Autodesk Fusion 360 part; units mm, degrees
note: some values were not read from the file. Chosen so that the rebuilt part matches the saved one: which face or edge a step refers to. Set by a fixed rule: which sketch regions a step uses.
(part 2 of 2)
sketch "Sketch4" plane through (20.4456, 0, 0) normal (1, 0, 0) x (0, 0, -1)
  arc A0 (20.4324, 154.945) -> (19.9602, 157.428) centre (20.32, 156.21) ccw
  arc A1 (19.9602, 157.428) -> (20.4324, 154.945) centre (20.0726, 156.1629) ccw
  circle A2 centre (21.6948, 142.2077) radius 3.175
  line L0 (12.648, 144.8633) -> (12.648, 132.4457)
  line L1 (12.648, 132.4457) -> (10.108, 132.4457)
  line L2 (10.108, 132.4457) -> (10.108, 144.8633)
  line L3 (10.108, 144.8633) -> (12.648, 144.8633)
  line L4 (-81.332, 144.78) -> (-78.792, 144.78)
  line L5 (-78.792, 144.78) -> (-78.792, 138.684)
  line L6 (-78.792, 138.684) -> (-81.332, 138.684)
  line L7 (-81.332, 138.684) -> (-81.332, 144.78)
  circle A3 centre (-84.1517, 161.0274) radius 3.175
  circle A4 centre (24.5119, 159.7522) radius 3.175
  arc A5 (-20.372, 13.97) -> (-12.752, 6.35) centre (-12.752, 13.97) ccw
  line L8 (-20.372, 13.97) -> (-20.372, 54.61)
  arc A6 (-20.372, 54.61) -> (-27.992, 62.23) centre (-27.992, 54.61) ccw
  line L9 (-27.992, 62.23) -> (-41.962, 62.23)
  arc A7 (-49.582, 69.85) -> (-41.962, 62.23) centre (-41.962, 69.85) ccw
  line L10 (-49.582, 69.85) -> (-49.582, 113.03)
  arc A8 (-41.962, 120.65) -> (-49.582, 113.03) centre (-41.962, 113.03) ccw
  line L11 (-41.962, 120.65) -> (-27.992, 120.65)
  arc A9 (-27.992, 120.65) -> (-20.372, 128.27) centre (-27.992, 128.27) ccw
  line L12 (-20.372, 128.27) -> (-20.372, 132.08)
  arc A10 (-12.752, 139.7) -> (-20.372, 132.08) centre (-12.752, 132.08) ccw
  line L13 (-12.752, 139.7) -> (-1.322, 139.7)
  arc A11 (6.298, 132.08) -> (-1.322, 139.7) centre (-1.322, 132.08) ccw
  line L14 (6.298, 132.08) -> (6.298, 13.97)
  arc A12 (-1.322, 6.35) -> (6.298, 13.97) centre (-1.322, 13.97) ccw
  line L15 (-1.322, 6.35) -> (-12.752, 6.35)
  line L16 (-18.467, 0) -> (-18.467, -2.54)
  line L17 (-18.467, -2.54) -> (3.4968, -2.54)
  line L18 (3.4968, -2.54) -> (3.4968, -10.16)
  line L19 (3.4968, -10.16) -> (10.108, -10.16)
  line L20 (10.108, -10.16) -> (10.108, -2.54)
  line L21 (10.108, -2.54) -> (12.648, -2.54)
  line L22 (12.648, -2.54) -> (12.648, -10.16)
  line L23 (12.648, -10.16) -> (20.32, -10.16)
  line L24 (20.32, -10.16) -> (20.32, 124.46)
  line L25 (20.32, 124.46) -> (30.428, 124.46)
  line L26 (30.428, 124.46) -> (30.428, 165.1009)
  line L27 (30.428, 165.1009) -> (17.232, 165.1009)
  arc A13 (18.014, 152.4) -> (17.232, 165.1009) centre (-85.5242, 152.4) ccw
  line L28 (18.014, 152.4) -> (-21.642, 152.4)
  line L29 (-21.642, 152.4) -> (-21.642, 145.288)
  line L30 (-21.642, 145.288) -> (-24.182, 145.288)
  line L31 (-24.182, 145.288) -> (-24.182, 152.4)
  line L32 (-24.182, 152.4) -> (-81.332, 152.4)
  line L33 (-81.332, 152.4) -> (-81.332, 152.4009)
  line L34 (-81.332, 152.4009) -> (-86.7309, 152.4009)
  line L35 (-86.7309, 152.4009) -> (-87.0413, 154.9409)
  line L36 (-87.0413, 154.9409) -> (-73.712, 156.5697)
  line L37 (-73.712, 156.5697) -> (-73.712, 166.37)
  line L38 (-73.712, 166.37) -> (-94.032, 166.37)
  line L39 (-94.032, 166.37) -> (-94.032, 127.3528)
  line L40 (-94.032, 127.3528) -> (-81.332, 127.3528)
  line L41 (-81.332, 127.3528) -> (-81.332, 12.7)
  line L42 (-81.332, 12.7) -> (-91.44, 12.7)
  line L43 (-91.44, 12.7) -> (-91.44, -10.16)
  line L44 (-91.44, -10.16) -> (-81.332, -10.16)
  line L45 (-81.332, -10.16) -> (-81.332, -2.54)
  line L46 (-81.332, -2.54) -> (-78.792, -2.54)
  line L47 (-78.792, -2.54) -> (-78.792, -10.16)
  line L48 (-78.792, -10.16) -> (-63.5, -10.16)
  line L49 (-63.5, -10.16) -> (-63.5, -2.54)
  line L50 (-63.5, -2.54) -> (-34.215, -2.54)
  line L51 (-34.215, -2.54) -> (-34.215, 0)
  line L52 (-34.215, 0) -> (-18.467, 0)
  arc A14 (20.4324, 154.945) -> (19.9602, 157.428) centre (20.32, 156.21) ccw
  arc A15 (19.9602, 157.428) -> (20.4324, 154.945) centre (20.0726, 156.1629) ccw
  circle A16 centre (21.6948, 142.2077) radius 3.175
  line L53 (12.648, 132.4457) -> (12.648, 144.8633)
  line L54 (12.648, 144.8633) -> (10.108, 144.8633)
  line L55 (10.108, 144.8633) -> (10.108, 132.4457)
  line L56 (10.108, 132.4457) -> (12.648, 132.4457)
  line L57 (-78.792, 144.78) -> (-81.332, 144.78)
  line L58 (-81.332, 144.78) -> (-81.332, 138.684)
  line L59 (-81.332, 138.684) -> (-78.792, 138.684)
  line L60 (-78.792, 138.684) -> (-78.792, 144.78)
  circle A17 centre (-84.1517, 161.0274) radius 3.175
  circle A18 centre (24.5119, 159.7522) radius 3.175
  arc A19 (-20.372, 13.97) -> (-12.752, 6.35) centre (-12.752, 13.97) ccw
  line L61 (-12.752, 6.35) -> (-1.322, 6.35)
  arc A20 (-1.322, 6.35) -> (6.298, 13.97) centre (-1.322, 13.97) ccw
  line L62 (6.298, 13.97) -> (6.298, 132.08)
  arc A21 (6.298, 132.08) -> (-1.322, 139.7) centre (-1.322, 132.08) ccw
  line L63 (-1.322, 139.7) -> (-12.752, 139.7)
  arc A22 (-12.752, 139.7) -> (-20.372, 132.08) centre (-12.752, 132.08) ccw
  line L64 (-20.372, 132.08) -> (-20.372, 128.27)
  arc A23 (-27.992, 120.65) -> (-20.372, 128.27) centre (-27.992, 128.27) ccw
  line L65 (-27.992, 120.65) -> (-41.962, 120.65)
  arc A24 (-41.962, 120.65) -> (-49.582, 113.03) centre (-41.962, 113.03) ccw
  line L66 (-49.582, 113.03) -> (-49.582, 69.85)
  arc A25 (-49.582, 69.85) -> (-41.962, 62.23) centre (-41.962, 69.85) ccw
  line L67 (-41.962, 62.23) -> (-27.992, 62.23)
  arc A26 (-20.372, 54.61) -> (-27.992, 62.23) centre (-27.992, 54.61) ccw
  line L68 (-20.372, 54.61) -> (-20.372, 13.97)
  line L69 (-18.467, -2.54) -> (-18.467, 0)
  line L70 (-18.467, 0) -> (-34.215, 0)
  line L71 (-34.215, 0) -> (-34.215, -2.54)
  line L72 (-34.215, -2.54) -> (-63.5, -2.54)
  line L73 (-63.5, -2.54) -> (-63.5, -10.16)
  line L74 (-63.5, -10.16) -> (-78.792, -10.16)
  line L75 (-78.792, -10.16) -> (-78.792, -2.54)
  line L76 (-78.792, -2.54) -> (-81.332, -2.54)
  line L77 (-81.332, -2.54) -> (-81.332, -10.16)
  line L78 (-81.332, -10.16) -> (-91.44, -10.16)
  line L79 (-91.44, -10.16) -> (-91.44, 12.7)
  line L80 (-91.44, 12.7) -> (-81.332, 12.7)
  line L81 (-81.332, 12.7) -> (-81.332, 127.3528)
  line L82 (-81.332, 127.3528) -> (-94.032, 127.3528)
  line L83 (-94.032, 127.3528) -> (-94.032, 166.37)
  line L84 (-94.032, 166.37) -> (-73.712, 166.37)
  line L85 (-73.712, 166.37) -> (-73.712, 156.5697)
  line L86 (-73.712, 156.5697) -> (-87.0413, 154.9409)
  line L87 (-87.0413, 154.9409) -> (-86.7309, 152.4009)
  line L88 (-86.7309, 152.4009) -> (-81.332, 152.4009)
  line L89 (-81.332, 152.4009) -> (-81.332, 152.4)
  line L90 (-81.332, 152.4) -> (-24.182, 152.4)
  line L91 (-24.182, 152.4) -> (-24.182, 145.288)
  line L92 (-24.182, 145.288) -> (-21.642, 145.288)
  line L93 (-21.642, 145.288) -> (-21.642, 152.4)
  line L94 (-21.642, 152.4) -> (18.014, 152.4)
  arc A27 (18.014, 152.4) -> (17.232, 165.1009) centre (-85.5242, 152.4) ccw
  line L95 (17.232, 165.1009) -> (30.428, 165.1009)
  line L96 (30.428, 165.1009) -> (30.428, 124.46)
  line L97 (30.428, 124.46) -> (20.32, 124.46)
  line L98 (20.32, 124.46) -> (20.32, -10.16)
  line L99 (20.32, -10.16) -> (12.648, -10.16)
  line L100 (12.648, -10.16) -> (12.648, -2.54)
  line L101 (12.648, -2.54) -> (10.108, -2.54)
  line L102 (10.108, -2.54) -> (10.108, -10.16)
  line L103 (10.108, -10.16) -> (3.4968, -10.16)
  line L104 (3.4968, -10.16) -> (3.4968, -2.54)
  line L105 (3.4968, -2.54) -> (-18.467, -2.54)
  line L106 (-68.58, 144.78) -> (-58.42, 144.78)
  line L107 (-58.42, 144.78) -> (-58.42, 152.4)
  line L108 (-58.42, 152.4) -> (-68.58, 152.4)
  line L109 (-68.58, 152.4) -> (-68.58, 144.78)
  line L110 (-38.1, 144.78) -> (-30.48, 144.78)
  line L111 (-30.48, 144.78) -> (-30.48, 152.4)
  line L112 (-30.48, 152.4) -> (-38.1, 152.4)
  line L113 (-38.1, 152.4) -> (-38.1, 144.78)
  line L114 (3.3659, 148.59) -> (10.108, 148.59)
  line L115 (10.108, 148.59) -> (10.108, 152.4)
  line L116 (10.108, 152.4) -> (3.3659, 152.4)
  line L117 (3.3659, 152.4) -> (3.3659, 148.59)
  point P0 (10.108, 152.4)
extrude "Extrude4'" cut sketch "Sketch4" against normal blind 2.54 contours L28 L94 L114 L115 L116 L117 | L32 L90 L110 L111 L112 L113 | L32 L90 L106 L107 L108 L109 bodies 6 in component "right"
sketch "Sketch5" plane through (0, 0, -12.648) normal (0, 0, -1) x (-1, 0, 0)
  line L0 (39.2444, -2.54) -> (39.2444, 0)
  line L1 (39.2444, 0) -> (49.4044, 0)
  line L2 (49.4044, 0) -> (49.4044, -2.54)
  line L3 (49.4044, -2.54) -> (39.2444, -2.54)
  line L4 (-9.7776, -2.54) -> (-9.7776, 0)
  line L5 (-9.7776, 0) -> (3.4304, 0)
  line L6 (3.4304, 0) -> (3.4304, -2.54)
  line L7 (3.4304, -2.54) -> (-9.7776, -2.54)
  line L8 (64.6444, -2.54) -> (64.6444, 132.4457)
  line L9 (64.6444, 132.4457) -> (69.7244, 132.4457)
  line L10 (69.7244, 132.4457) -> (69.7244, 144.7757)
  arc A0 (69.7244, 144.7757) -> (64.6444, 144.8633) centre (64.6444, -2.54) ccw
  line L11 (64.6444, 144.8633) -> (64.6444, 152.4)
  line L12 (64.6444, 152.4) -> (-17.9056, 152.4)
  line L13 (-17.9056, 152.4) -> (-17.9056, 144.8633)
  arc A1 (-17.9056, 144.8633) -> (-22.9856, 144.7757) centre (-17.9056, -2.54) ccw
  line L14 (-22.9856, 144.7757) -> (-22.9856, 132.4457)
  line L15 (-22.9856, 132.4457) -> (-17.9056, 132.4457)
  line L16 (-17.9056, 132.4457) -> (-17.9056, -2.54)
  line L17 (-17.9056, -2.54) -> (-20.4456, -2.54)
  line L18 (-20.4456, -2.54) -> (-20.7288, 7.6202)
  line L19 (-20.7288, 7.6202) -> (-24.3812, 7.6202)
  line L20 (-24.3812, 7.6202) -> (-24.3812, -10.16)
  line L21 (-24.3812, -10.16) -> (71.12, -10.16)
  line L22 (71.12, -10.16) -> (71.12, 7.6202)
  line L23 (71.12, 7.6202) -> (67.4676, 7.6202)
  line L24 (67.4676, 7.6202) -> (67.1844, -2.54)
  line L25 (67.1844, -2.54) -> (64.6444, -2.54)
  line L26 (-9.8069, 146.05) -> (-2.54, 146.05)
  line L27 (-2.54, 146.05) -> (-2.54, 152.4)
  line L28 (-2.54, 152.4) -> (-9.8069, 152.4)
  line L29 (-9.8069, 152.4) -> (-9.8069, 146.05)
  line L30 (12.1172, 146.05) -> (17.78, 146.05)
  line L31 (17.78, 146.05) -> (17.78, 152.4)
  line L32 (17.78, 152.4) -> (12.1172, 152.4)
  line L33 (12.1172, 152.4) -> (12.1172, 146.05)
  line L34 (-17.9056, 152.4) -> (64.6444, 152.4)
  line L35 (40.7725, 146.05) -> (50.8, 146.05)
  line L36 (50.8, 146.05) -> (50.8, 152.4)
  line L37 (50.8, 152.4) -> (40.7725, 152.4)
  line L38 (40.7725, 152.4) -> (40.7725, 146.05)
extrude "Extrude2''" cut sketch "Sketch5" against normal blind 2.54 contours L12 L34 L35 L36 L37 L38 | L12 L30 L31 L32 L33 L34 | L12 L26 L27 L28 L29 L34 bodies 3 in component "back"
sketch "Sketch6" plane through (-67.1844, 0, 0) normal (-1, 0, 0) x (0, 0, 1)
  circle A0 centre (-24.5119, 159.7522) radius 3.175
  circle A1 centre (-21.6948, 142.2077) radius 3.175
  circle A2 centre (-20.32, 156.21) radius 1.27
  line L0 (78.792, 144.78) -> (81.332, 144.78)
  line L1 (81.332, 144.78) -> (81.332, 138.684)
  line L2 (81.332, 138.684) -> (78.792, 138.684)
  line L3 (78.792, 138.684) -> (78.792, 144.78)
  circle A3 centre (84.1517, 161.0274) radius 3.175
  line L4 (-12.648, 132.4457) -> (-12.648, 144.8633)
  line L5 (-12.648, 144.8633) -> (-10.108, 144.8633)
  line L6 (-10.108, 144.8633) -> (-10.108, 132.4457)
  line L7 (-10.108, 132.4457) -> (-12.648, 132.4457)
  line L8 (81.332, -2.54) -> (81.332, -10.16)
  line L9 (81.332, -10.16) -> (91.44, -10.16)
  line L10 (91.44, -10.16) -> (91.44, 12.7)
  line L11 (91.44, 12.7) -> (81.332, 12.7)
  line L12 (81.332, 12.7) -> (81.332, 127.3528)
  line L13 (81.332, 127.3528) -> (94.032, 127.3528)
  line L14 (94.032, 127.3528) -> (94.032, 166.37)
  line L15 (94.032, 166.37) -> (73.712, 166.37)
  line L16 (73.712, 166.37) -> (73.712, 156.5697)
  line L17 (73.712, 156.5697) -> (87.0413, 154.9409)
  line L18 (87.0413, 154.9409) -> (86.7309, 152.4009)
  line L19 (86.7309, 152.4009) -> (81.332, 152.4009)
  line L20 (81.332, 152.4009) -> (81.332, 152.4)
  line L21 (81.332, 152.4) -> (24.182, 152.4)
  line L22 (24.182, 152.4) -> (24.182, 145.288)
  line L23 (24.182, 145.288) -> (21.642, 145.288)
  line L24 (21.642, 145.288) -> (21.642, 152.4)
  line L25 (21.642, 152.4) -> (-18.014, 152.4)
  arc A4 (-17.232, 165.1009) -> (-18.014, 152.4) centre (85.5242, 152.4) ccw
  line L26 (-17.232, 165.1009) -> (-30.428, 165.1009)
  line L27 (-30.428, 165.1009) -> (-30.428, 124.46)
  line L28 (-30.428, 124.46) -> (-12.648, 124.46)
  line L29 (-12.648, 124.46) -> (-12.648, 10.16)
  line L30 (-12.648, 10.16) -> (-20.32, 10.16)
  line L31 (-20.32, 10.16) -> (-20.32, -10.16)
  line L32 (-20.32, -10.16) -> (-12.648, -10.16)
  line L33 (-12.648, -10.16) -> (-12.648, -2.54)
  line L34 (-12.648, -2.54) -> (-10.108, -2.54)
  line L35 (-10.108, -2.54) -> (-10.108, -10.16)
  line L36 (-10.108, -10.16) -> (-3.4968, -10.16)
  line L37 (-3.4968, -10.16) -> (-3.4968, -2.54)
  line L38 (-3.4968, -2.54) -> (63.5, -2.54)
  line L39 (63.5, -2.54) -> (63.5, -10.16)
  line L40 (63.5, -10.16) -> (78.792, -10.16)
  line L41 (78.792, -10.16) -> (78.792, -2.54)
  line L42 (78.792, -2.54) -> (81.332, -2.54)
  line L43 (0.3486, 145.1838) -> (11.7805, 145.1838)
  line L44 (11.7805, 145.1838) -> (11.7805, 152.4)
  line L45 (11.7805, 152.4) -> (0.3486, 152.4)
  line L46 (0.3486, 152.4) -> (0.3486, 145.1838)
  line L47 (30.48, 144.78) -> (38.1, 144.78)
  line L48 (38.1, 144.78) -> (38.1, 152.4)
  line L49 (38.1, 152.4) -> (30.48, 152.4)
  line L50 (30.48, 152.4) -> (30.48, 144.78)
  line L51 (58.42, 144.78) -> (68.58, 144.78)
  line L52 (68.58, 144.78) -> (68.58, 152.4)
  line L53 (68.58, 152.4) -> (58.42, 152.4)
  line L54 (58.42, 152.4) -> (58.42, 144.78)
  point P0 (0.3486, 145.1838)
  point P1 (11.7805, 152.4)
  point P2 (30.48, 144.78)
  point P3 (38.1, 152.4)
  point P4 (58.42, 144.78)
  point P5 (68.58, 152.4)
extrude "Extrude4''" cut sketch "Sketch6" against normal blind 2.54 contours L21 L51 L52 L53 L54 | L21 L47 L48 L49 L50 | L25 L43 L44 L45 L46 bodies 5 in component "left"
sketch "Sketch7" plane through (0, 0, 81.332) normal (0, 0, 1) x (1, 0, 0)
  line L0 (-53.4684, 0) -> (-43.3084, 0)
  line L1 (-43.3084, 0) -> (-43.3084, -2.54)
  line L2 (-43.3084, -2.54) -> (-53.4684, -2.54)
  line L3 (-53.4684, -2.54) -> (-53.4684, 0)
  line L4 (-1.3984, 0) -> (10.7936, 0)
  line L5 (10.7936, 0) -> (10.7936, -2.54)
  line L6 (10.7936, -2.54) -> (-1.3984, -2.54)
  line L7 (-1.3984, -2.54) -> (-1.3984, 0)
  line L8 (-71.12, -10.16) -> (24.3812, -10.16)
  line L9 (24.3812, -10.16) -> (24.3812, 7.6202)
  line L10 (24.3812, 7.6202) -> (20.7288, 7.6202)
  line L11 (20.7288, 7.6202) -> (20.4456, -2.54)
  line L12 (20.4456, -2.54) -> (17.9056, -2.54)
  line L13 (17.9056, -2.54) -> (17.9056, 138.684)
  line L14 (17.9056, 138.684) -> (21.842, 138.684)
  line L15 (21.842, 138.684) -> (21.842, 144.7274)
  arc A0 (21.842, 144.7274) -> (17.9056, 144.78) centre (17.9056, -2.54) ccw
  line L16 (17.9056, 144.78) -> (17.9056, 152.4)
  line L17 (17.9056, 152.4) -> (-64.6444, 152.4)
  line L18 (-64.6444, 152.4) -> (-64.6444, 144.78)
  arc A1 (-64.6444, 144.78) -> (-68.5808, 144.7274) centre (-64.6444, -2.54) ccw
  line L19 (-68.5808, 144.7274) -> (-68.5808, 138.684)
  line L20 (-68.5808, 138.684) -> (-64.6444, 138.684)
  line L21 (-64.6444, 138.684) -> (-64.6444, -2.54)
  line L22 (-64.6444, -2.54) -> (-67.1844, -2.54)
  line L23 (-67.1844, -2.54) -> (-67.4676, 7.6202)
  line L24 (-67.4676, 7.6202) -> (-71.12, 7.6202)
  line L25 (-71.12, 7.6202) -> (-71.12, -10.16)
  line L26 (-57.028, 144.7274) -> (-45.72, 144.7274)
  line L27 (-45.72, 144.7274) -> (-45.72, 152.4)
  line L28 (-45.72, 152.4) -> (-57.028, 152.4)
  line L29 (-57.028, 152.4) -> (-57.028, 144.7274)
  line L30 (-35.3043, 144.7274) -> (-30.48, 144.7274)
  line L31 (-30.48, 144.7274) -> (-30.48, 152.4)
  line L32 (-30.48, 152.4) -> (-35.3043, 152.4)
  line L33 (-35.3043, 152.4) -> (-35.3043, 144.7274)
  line L34 (-5.0802, 144.7274) -> (2.54, 144.7274)
  line L35 (2.54, 144.7274) -> (2.54, 152.4)
  line L36 (2.54, 152.4) -> (-5.0802, 152.4)
  line L37 (-5.0802, 152.4) -> (-5.0802, 144.7274)
  point P0 (2.54, 152.4)
extrude "Extrude2'''" cut sketch "Sketch7" against normal blind 2.54 contours L17 L26 L27 L28 L29 | L17 L34 L35 L36 L37 | L17 L30 L31 L32 L33 bodies 2 in component "front"
sketch "Sketch8" plane through (0, -2.54, 0) normal (0, -1, 0) x (1, 0, 0)
  line L0 (-7.2404, 27.484) -> (6.9836, 27.484)
  line L1 (6.9836, 27.484) -> (6.9836, 24.436)
  line L2 (6.9836, 24.436) -> (-7.2404, 24.436)
  line L3 (-7.2404, 24.436) -> (-7.2404, 27.484)
  line L4 (12.7, 0) -> (12.7, -5.08)
  line L5 (12.7, -5.08) -> (-2.54, -5.08)
  line L6 (-2.54, -5.08) -> (-2.54, 0)
  line L7 (-2.54, 0) -> (12.7, 0)
  circle A0 centre (-25.0204, 34.723) radius 8.73
  line L8 (20.6996, 29.897) -> (23.8746, 29.897)
  line L9 (23.8746, 29.897) -> (23.8746, 22.785)
  line L10 (23.8746, 22.785) -> (20.6996, 22.785)
  line L11 (20.6996, 22.785) -> (20.6996, 29.897)
  line L12 (-56.5164, 21.642) -> (-56.5164, 24.182)
  line L13 (-56.5164, 24.182) -> (-45.3404, 24.182)
  line L14 (-45.3404, 24.182) -> (-45.3404, 21.642)
  line L15 (-45.3404, 21.642) -> (-56.5164, 21.642)
  line L16 (-20.7024, 21.642) -> (-20.7024, 24.182)
  line L17 (-20.7024, 24.182) -> (-12.5744, 24.182)
  line L18 (-12.5744, 24.182) -> (-12.5744, 21.642)
  line L19 (-12.5744, 21.642) -> (-20.7024, 21.642)
  line L20 (-3.4304, -10.108) -> (-3.4304, -15.188)
  line L21 (-3.4304, -15.188) -> (9.7776, -15.188)
  line L22 (9.7776, -15.188) -> (9.7776, -10.108)
  line L23 (9.7776, -10.108) -> (17.9056, -10.108)
  line L24 (17.9056, -10.108) -> (17.9056, 18.467)
  line L25 (17.9056, 18.467) -> (27.6846, 18.467)
  line L26 (27.6846, 18.467) -> (27.6846, 34.215)
  line L27 (27.6846, 34.215) -> (17.9056, 34.215)
  line L28 (17.9056, 34.215) -> (17.9056, 78.792)
  line L29 (17.9056, 78.792) -> (10.7936, 78.792)
  line L30 (10.7936, 78.792) -> (10.7936, 83.872)
  line L31 (10.7936, 83.872) -> (-1.3984, 83.872)
  line L32 (-1.3984, 83.872) -> (-1.3984, 78.792)
  line L33 (-1.3984, 78.792) -> (-43.3084, 78.792)
  line L34 (-43.3084, 78.792) -> (-43.3084, 83.872)
  line L35 (-43.3084, 83.872) -> (-53.4684, 83.872)
  line L36 (-53.4684, 83.872) -> (-53.4684, 78.792)
  line L37 (-53.4684, 78.792) -> (-57.0244, 78.792)
  arc A1 (-57.0244, 78.792) -> (-64.6444, 71.172) centre (-57.0244, 71.172) ccw
  line L38 (-64.6444, 71.172) -> (-64.6444, -10.108)
  line L39 (-64.6444, -10.108) -> (-49.4044, -10.108)
  line L40 (-49.4044, -10.108) -> (-49.4044, -15.188)
  line L41 (-49.4044, -15.188) -> (-39.2444, -15.188)
  line L42 (-39.2444, -15.188) -> (-39.2444, -10.108)
  line L43 (-39.2444, -10.108) -> (-3.4304, -10.108)
  line L44 (-60.96, 68.58) -> (-64.6444, 68.58)
  line L45 (-64.6444, 68.58) -> (-64.6444, 63.5)
  line L46 (-64.6444, 63.5) -> (-60.96, 63.5)
  line L47 (-60.96, 63.5) -> (-60.96, 68.58)
  line L48 (-60.96, 49.728) -> (-64.6444, 49.728)
  line L49 (-64.6444, 49.728) -> (-64.6444, 41.5831)
  line L50 (-64.6444, 41.5831) -> (-60.96, 41.5831)
  line L51 (-60.96, 41.5831) -> (-60.96, 49.728)
  line L52 (-60.96, 30.532) -> (-64.6444, 30.532)
  line L53 (-64.6444, 30.532) -> (-64.6444, 24.182)
  line L54 (-64.6444, 24.182) -> (-60.96, 24.182)
  line L55 (-60.96, 24.182) -> (-60.96, 30.532)
  line L56 (-60.96, 15.24) -> (-64.6444, 15.24)
  line L57 (-64.6444, 15.24) -> (-64.6444, 11.7805)
  line L58 (-64.6444, 11.7805) -> (-60.96, 11.7805)
  line L59 (-60.96, 11.7805) -> (-60.96, 15.24)
  line L60 (-60.96, -5.08) -> (-64.6444, -5.08)
  line L61 (-64.6444, -5.08) -> (-64.6444, -10.108)
  line L62 (-64.6444, -10.108) -> (-60.96, -10.108)
  line L63 (-60.96, -10.108) -> (-60.96, -5.08)
  line L64 (-36.9333, -5.08) -> (-31.3436, -5.08)
  line L65 (-31.3436, -5.08) -> (-31.3436, -10.108)
  line L66 (-31.3436, -10.108) -> (-36.9333, -10.108)
  line L67 (-36.9333, -10.108) -> (-36.9333, -5.08)
  line L68 (-12.7, -5.08) -> (-6.7491, -5.08)
  line L69 (-6.7491, -5.08) -> (-6.7491, -10.108)
  line L70 (-6.7491, -10.108) -> (-12.7, -10.108)
  line L71 (-12.7, -10.108) -> (-12.7, -5.08)
  line L72 (12.7, 15.24) -> (17.9056, 15.24)
  line L73 (17.9056, 15.24) -> (17.9056, 9.1381)
  line L74 (17.9056, 9.1381) -> (12.7, 9.1381)
  line L75 (12.7, 9.1381) -> (12.7, 15.24)
  line L76 (17.9056, 21.642) -> (17.9056, -3.3659)
  line L77 (12.7, 45.72) -> (17.9056, 45.72)
  line L78 (17.9056, 45.72) -> (17.9056, 38.1)
  line L79 (17.9056, 38.1) -> (12.7, 38.1)
  line L80 (12.7, 38.1) -> (12.7, 45.72)
  line L81 (12.7, 71.12) -> (17.9056, 71.12)
  line L82 (17.9056, 71.12) -> (17.9056, 78.792)
  line L83 (17.9056, 78.792) -> (12.7, 78.792)
  line L84 (12.7, 78.792) -> (12.7, 71.12)
  line L85 (-10.16, 73.66) -> (-25.4346, 73.66)
  line L86 (-25.4346, 73.66) -> (-25.4346, 78.792)
  line L87 (-25.4346, 78.792) -> (-10.16, 78.792)
  line L88 (-10.16, 78.792) -> (-10.16, 73.66)
  point P0 (-64.6444, 63.5)
  point P1 (-64.6444, 24.182)
  point P2 (-64.6444, 11.7805)
  point P3 (17.9056, 38.1)
extrude "Extrude1''''''" cut sketch "Sketch8" against normal blind 2.54 contours L43 L68 L69 L70 L71 | L43 L64 L65 L66 L67 | L24 L72 L73 L74 L75 L76 | L38 L39 L60 L61 L62 L63 | L28 L77 L78 L79 L80 | L38 L56 L57 L58 L59 | L28 L29 L81 L82 L83 L84 | L38 L48 L49 L50 L51 | L38 L44 L45 L46 L47 | L33 L85 L86 L87 L88 bodies 10 in component "floorfromorig"
component "front" placed x (1, 0, 0) y (0, 1, 0) z (0, 0, 1) at (0, 0, 0)
component "back" placed x (1, 0, 0) y (0, 1, 0) z (0, 0, 1) at (0, 0, 0)
component "midwall" placed x (1, 0, 0) y (0, 1, 0) z (0, 0, 1) at (0, 0, 0)
component "left" placed x (1, 0, 0) y (0, 1, 0) z (0, 0, 1) at (0, 0, 0)
component "right" placed x (1, 0, 0) y (0, 1, 0) z (0, 0, 1) at (0, 0, 0)
component "top" placed x (1, 0, 0) y (0, 1, 0) z (0, 0, 1) at (0, 0, 0)
component "door (1)" placed x (1, 0, 0) y (0, 1, 0) z (0, 0, 1) at (0, 0, 0)
component "door" placed x (1, 0, 0) y (0, 1, 0) z (0, 0, 1) at (0, 0, 0)
component "roof" placed x (1, 0, 0) y (0, 1, 0) z (0, 0, 1) at (0, 0, 0)
component "floorfromorig" placed x (1, 0, 0) y (0, 1, 0) z (0, 0, 1) at (0, 0, 0)
equation "w = 3.25 in" comment "inner width"
equation "d = 3.5 in" comment "inner depth"
equation "h = 6 in" comment "inner height"
equation "t = 0.1 in" comment "material thickness"
equation "d13 = t"
equation "d14 = t"
equation "d15 = t * 1.25"
equation "d16 = t * 1.1"
equation "d17 = d"
equation "d18 = t * 1.5"
equation "d19 = t * 2"
equation "d20 = t * 2"
equation "d21 = w"
equation "d22 = slot * 1.1"
equation "slot = 0.4 in" comment "typical slot/tab length"
equation "d24 = slot * 1.0"
equation "d25 = slot * 1.2"
equation "d26 = slot * 0.7"
equation "d27 = slot * 1.1"
equation "d28 = slot * 0.8"
equation "d29 = slot * 3"
equation "d30 = slot * 0.8"
equation "d31 = slot * 1.0"
equation "d32 = slot * 1.5"
equation "d33 = slot * 1.3"
equation "d34 = slot * 0.8"
equation "bcd = 1.25 in" comment "battery compartment depth"
equation "d36 = bcd"
equation "d37 = bcd * 0.9"
equation "d38 = t * 1.7"
equation "d39 = t * 1.7"
equation "d40 = slot * 0.7"
equation "d41 = -t"
equation "d46 = h"
equation "d50 = t"
equation "d51 = t"
equation "d52 = t"
equation "d54 = h"
equation "d55 = t * 2"
equation "d56 = t"
equation "d58 = w"
equation "d59 = h"
equation "d60 = t * 1.1"
equation "d61 = t * 2"
equation "d62 = slot * 0.7"
equation "ptfromleft = 1 in"
equation "ptwidth = 1.95 in" comment "long horiz dim of plantower"
equation "boardwid = 2.6 in" comment "width hole-hole of board"
equation "boardht = 1.8 in" comment "height hole-hole of board"
equation "boardfromr = 0.15 in" comment "board holes from right"
equation "d68 = boardfromr"
equation "d69 = boardht"
equation "d70 = boardwid"
equation "d71 = ptfromleft"
equation "d72 = ptwidth"
equation "tiehole = 0.10 in" comment "ctr board tie hole diam"
equation "ptmidht = 0.75 in" comment "midheight for plantower"
equation "d75 = ptmidht"
equation "d76 = tiehole"
equation "d77 = tiehole"
equation "d78 = tiehole"
equation "d79 = tiehole"
equation "d80 = tiehole"
equation "d81 = tiehole"
equation "d82 = ptfromleft"
equation "d83 = ptwidth"
equation "ptdepth = 0.83 in" comment "plantower depth (thickness)"
equation "ptcircrad = 0.3437 in" comment "plantower circle radius"
equation "ptcirclefromend = 0.56 in" comment "circle center from end"
equation "ptrectfromr = 0.13 in" comment "plantower rect from right"
equation "ptrectfromside = 0.01 in" comment "plantower rect from near side"
equation "ptrectlen = 0.56 in" comment "plantower rect length"
equation "ptrectw = 0.12 in" comment "width of plantower rect"
equation "d91 = ptdepth"
equation "d92 = ptcircrad * 2"
equation "d93 = ptcirclefromend"
equation "d94 = ptrectlen"
equation "d95 = ptrectfromr"
equation "d96 = ptrectfromside"
equation "d97 = ptrectw"
equation "d98 = t"
equation "d100 = t"
equation "d101 = hanghole"
equation "hanghole = 0.25 in" comment "hole for zip ties to hang"
equation "d103 = hanghole"
equation "d104 = tiehole"
equation "d105 = hanghole"
equation "d118 = t"
equation "d121 = t / 2"
equation "d123 = t * 2.5"
equation "eaves = 0.5 in"
equation "d126 = eaves"
equation "d127 = eaves"
equation "d128 = eaves"
equation "d129 = eaves"
equation "d133 = t * 2"
equation "d134 = t * 2"
equation "d139 = t"
equation "d141 = t"
equation "d150 = hanghole"
equation "d151 = t"
equation "d155 = t"
equation "d157 = t"
equation "d159 = t * 2.5"
equation "d160 = t"
equation "d161 = t"
equation "d162 = t * 0.8"
equation "d163 = t * 0.8"
equation "d164 = t * 0.8"
equation "d165 = t"
equation "d167 = -t"
equation "d169 = -t"
equation "d175 = -t"
equation "d177 = t + 0.5 * tiehole"
equation "d180 = -t"
equation "d182 = -t"
equation "d184 = -t"
equation "d186 = -t"
equation "d188 = -t"
